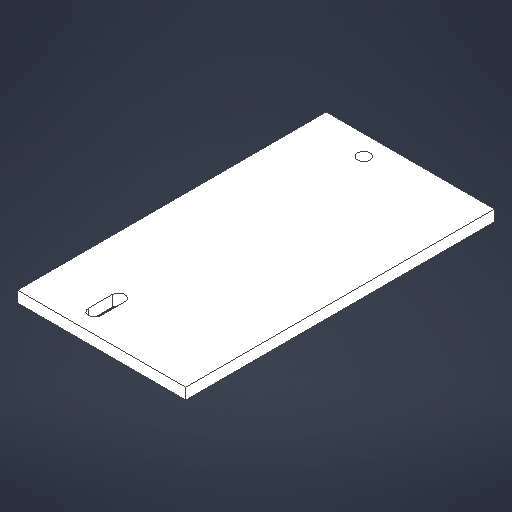
# Autodesk Inventor part: TapaBatería
Saved by Autodesk Inventor 2026.1 (Build 301233020, 233B)
## iProperties
Created: 2025-11-24
Part Number: TapaBatería
Material: Generic
Document SubType Name: Modeling
Designer: Tito Luyo Murata
Density: 1 g/cm^3
Appearance: Default
Author: Tito Luyo Murata
Autodesk Inventor part; units mm, degrees
ref_plane "YZ Plane" through (0, 0, 0) normal (1, 0, 0) x (0, 1, 0)
ref_plane "XZ Plane" through (0, 0, 0) normal (0, 1, 0) x (-1, 0, 0)
ref_plane "XY Plane" through (0, 0, 0) normal (0, 0, 1) x (1, 0, 0)
sketch "Sketch1" plane through (0, 0, 0) normal (0, 1, 0) x (-1, 0, 0)
  line L0 (0, 0) -> (42.5, 0)
  line L1 (42.5, 0) -> (42.5, -78)
  line L2 (42.5, -78) -> (0, -78)
  line L3 (0, -78) -> (0, 0)
  circle A0 centre (28, -73) radius 1.6
  line L4 (28, -3.4) -> (28, -3.4)
  line L5 (26.4, -5) -> (26.4, -11)
  line L6 (28, -12.6) -> (28, -12.6)
  line L7 (29.6, -11) -> (29.6, -5)
  arc A1 (28, -12.6) -> (29.6, -11) centre (28, -11) ccw
  arc A2 (26.4, -11) -> (28, -12.6) centre (28, -11) ccw
  arc A3 (28, -3.4) -> (26.4, -5) centre (28, -5) ccw
  arc A4 (29.6, -5) -> (28, -3.4) centre (28, -5) ccw
  point P0 (26.4, -12.6)
  point P1 (26.4, -3.4)
  point P2 (29.6, -12.6)
  point P3 (29.6, -8)
  point P4 (28, -3.4)
  point P5 (28, -12.6)
  dimension "d0" = 42.5
  dimension "d1" = 78
  dimension "d5" = 3.2
  dimension "d6" = 14.5
  dimension "d7" = 5
  dimension "d10" = 3.2
  dimension "d11" = 9.2
  dimension "d12" = 8
  dimension "d13" = 1.6
  dimension "d14" = 14.5
  constraints: 16 end point, 8 point on circle, 8 tangent, 6 point on line, 5 centre point, 4 parallel, 3 equal radius, 2 horizontal, 2 perpendicular, 1 coincident, 1 midpoint
  measures "d0" distance of L1.end L2.end
  measures "d1" distance of L0.end L1.end
  measures "d5" diameter of A0
  measures "d6" distance from line of A0.centre L1
  measures "d7" distance from line of L2 A0.centre
  measures "d10" distance of point (29.6, -12.6) point (26.4, -12.6)
  measures "d11" distance of point (26.4, -12.6) point (26.4, -3.4)
  measures "d12" distance from line of L0 point (29.6, -8)
  measures "d13" radius of A1
  measures "d14" distance from line of A3.centre L1
extrude "Extrusion1" add sketch "Sketch1" along normal blind 2.8
body "Solid1"
